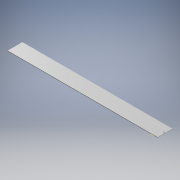
# Autodesk Inventor part: X-box-coverplate-2mm
Saved by Autodesk Inventor 2016 (Build 200138000, 138)
## iProperties
Created: 2015-04-22
Part Number: X-box-coverplate-2mm
Material: Aluminum 6061
Document SubType Name: Modeling
Designer: ax
Mass: 196.729 g
Surface Area: 753.468 cm^2
Volume: 72.8627 cm^3
Density: 2.7 g/cm^3
Appearance: Aluminum - Flat
Author: ax
Autodesk Inventor part; units mm, degrees
ref_plane "YZ Plane" through (0, 0, 0) normal (1, 0, 0) x (0, 1, 0)
ref_plane "XZ Plane" through (0, 0, 0) normal (0, 1, 0) x (-1, 0, 0)
ref_plane "XY Plane" through (0, 0, 0) normal (0, 0, 1) x (1, 0, 0)
ref_plane "Work Plane3" through (759.785, -2, 0) normal (0, 0, 1) x (-1, 0, 0)
sketch "Sketch2" plane through (759.785, -2, 0) normal (0, 0, 1) x (-1, 0, 0)
  line L0 (-16.8925, -4) -> (593.1075, -4)
  line L1 (593.1075, -4) -> (593.1075, 56)
  line L2 (593.1075, 56) -> (-16.8925, 56)
  line L3 (-16.8925, 56) -> (-16.8925, -4)
  point P0 (759.785, -2)
  dimension "d0" = 610
  dimension "d1" = 60
  constraints: 8 end point, 2 parallel, 1 horizontal, 1 perpendicular
  measures "d0" distance of L2.end L1.end
  measures "d1" distance of L1.end L0.end
extrude "Extrusion1" add sketch "Sketch2" along normal blind 2
sketch "Sketch4" plane through (759.785, -2, 2) normal (0, 0, 1) x (1, 0, 0)
  line L0 (16.8925, 4) -> (-593.1075, 4) projected
  line L1 (16.8925, -56) -> (16.8925, 4) projected
  point P0 (-759.785, 2)
  point P1 (11.8925, -26)
  point P2 (-288.1075, -26)
  point P3 (-588.1075, -26)
  dimension "d14" = 30
  dimension "d15" = 5
  dimension "d18" = 300
  constraints: 1 horizontal, 2 other
  measures "d14" distance from line of L0 point (11.893, -26)
  measures "d15" distance from line of L1 point (11.893, -26)
  measures "d18" distance of point (11.893, -26) point (-288.107, -26)
hole "Hole2" at (171.6775, -28, 2) at (471.6775, -28, 2) at (771.6775, -28, 2) direction (0, 0, -1) diameter 5 end through all
chamfer "Chamfer1" [suppressed]
sketch "Sketch5" plane through (759.785, -2, 2) normal (0, 0, 1) x (1, 0, 0)
  line L0 (16.8925, 4) -> (-593.1075, 4) projected
  line L1 (16.8925, -56) -> (16.8925, 4) projected
  point P0 (-13.1075, 1.5)
  point P1 (-63.1075, 1.5)
  point P2 (-113.1075, 1.5)
  point P3 (-163.1075, 1.5)
  point P4 (-213.1075, 1.5)
  point P5 (-263.1075, 1.5)
  point P6 (-313.1075, 1.5)
  point P7 (-363.1075, 1.5)
  point P8 (-413.1075, 1.5)
  point P9 (-463.1075, 1.5)
  point P10 (-513.1075, 1.5)
  point P11 (-563.1075, 1.5)
  point P12 (-13.1075, -53.5)
  point P13 (-63.1075, -53.5)
  point P14 (-113.1075, -53.5)
  point P15 (-163.1075, -53.5)
  point P16 (-213.1075, -53.5)
  point P17 (-263.1075, -53.5)
  point P18 (-313.1075, -53.5)
  point P19 (-363.1075, -53.5)
  point P20 (-413.1075, -53.5)
  point P21 (-463.1075, -53.5)
  point P22 (-513.1075, -53.5)
  point P23 (-563.1075, -53.5)
  dimension "d30" = 2.5
  dimension "d31" = 30
  dimension "d34" = 50
  dimension "d37" = 55
  constraints: 1 horizontal, 1 vertical, 23 other
  measures "d30" distance from line of L0 point (-13.107, 1.5)
  measures "d31" distance from line of L1 point (-13.107, 1.5)
  measures "d34" distance of point (-13.107, 1.5) point (-63.107, 1.5)
  measures "d37" distance of point (-13.107, 1.5) point (-13.107, -53.5)
hole "Hole3" at (646.6775, -55.5, 2) at (646.6775, -0.5, 2) at (596.6775, -0.5, 2) at (546.6775, -55.5, 2) at (546.6775, -0.5, 2) at (496.6775, -55.5, 2) at (496.6775, -0.5, 2) at (446.6775, -55.5, 2) at (446.6775, -0.5, 2) at (396.6775, -55.5, 2) at (396.6775, -0.5, 2) at (346.6775, -55.5, 2) at (346.6775, -0.5, 2) at (296.6775, -55.5, 2) at (296.6775, -0.5, 2) at (246.6775, -55.5, 2) at (246.6775, -0.5, 2) at (196.6775, -55.5, 2) at (196.6775, -0.5, 2) at (596.6775, -55.5, 2) at (746.6775, -55.5, 2) at (746.6775, -0.5, 2) at (696.6775, -55.5, 2) at (696.6775, -0.5, 2) direction (0, 0, -1) diameter 3 end through all
body "Solid1"
